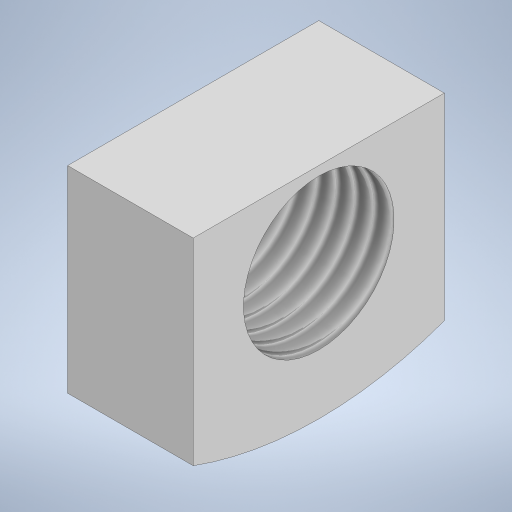
# Autodesk Inventor part: porta vite senza fine
Saved by Autodesk Inventor 2024 (Build 280153000, 153)
## iProperties
Created: 2024-03-01
Part Number: porta vite senza fine
Material: Generico
Document SubType Name: Modeling
Designer: Giorgio
Density: 1 g/cm^3
Appearance: Default
Author: Giorgio
Autodesk Inventor part; units mm, degrees
ref_plane "YZ Plane" through (0, 0, 0) normal (1, 0, 0) x (0, 1, 0)
ref_plane "XZ Plane" through (0, 0, 0) normal (0, 1, 0) x (-1, 0, 0)
ref_plane "XY Plane" through (0, 0, 0) normal (0, 0, 1) x (1, 0, 0)
sketch "Schizzo1" plane through (0, 0, 0) normal (1, 0, 0) x (0, 1, 0)
  line L0 (2.5344, 4.1858) -> (-5.3178, 4.1858)
  line L1 (-5.3178, -5.8142) -> (2.5344, -5.8142)
  line L2 (2.5344, -5.8142) -> (2.5344, 4.1858)
  circle A0 centre (-0.8257, -0.8142) radius 3
  line L3 (2.5344, 4.1858) -> (2.5344, -0.8142)
  arc A1 (-5.3178, 4.1858) -> (-5.3178, -5.8142) centre (8.3421, -0.8142) ccw
  point P0 (0, 0)
  dimension "d0" = 10
  dimension "d1" = 6
  constraints: 8 end point, 2 centre point, 2 point on circle, 1 horizontal, 1 midpoint, 1 parallel
  measures "d0" distance of L1.end L0.start
  measures "d1" diameter of A0
extrude "Estrusione1" add sketch "Schizzo1" against normal blind 5
thread "Filettatura1" size "M6x0.75" class "6H" standard "ANSI Metric M Profile" full length
